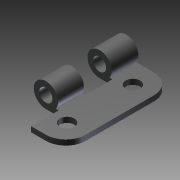
# Autodesk Inventor part: SHHPS5-2-pin
Saved by Autodesk Inventor 2015 SP1 (Build 190203100, 203)
## iProperties
Category: PARTsolutions
Company: MISUMI
Created: 2015-01-26
Part Number: SHHPS5-2-pin
Catalog Web Link: www.cadenas.de
Description: SHHPS,SHHPSD, SHHPT-pin-Stainless Steel Hinges, Steel Hinges
Vendor: MISUMI
Document SubType Name: Modeling
Designer: PARTuser1
Manufacturer: MISUMI
Mass: 1.95917 g
Surface Area: 22.9373 cm^2
Volume: 1.95917 cm^3
Density: 1 g/cm^3
Material: Generic
Appearance: PSOLRGB-192-192-192
PSOL_IDENT_0: {\\10.0.0.236\data_v8\23d-libs\misumi\metric\39_accessories_for_al_extrusions\shhps_r.prj},194 {VTYP=
PSOL_IDENT_1: 3D},{NB=SHHPS5-2-pin},{LINA=SHHPS5-2-pin},{NN=SHHPS,SHHPSD, SHHPT-pin},{DATE=17.11.2014 05:31:35},{G
PSOL_IDENT_2: EOMDATE=13.05.2009 09:15:00},{VERSION=},{LINEID=10},{LINESUBID=-1},{WBVAR=TS,NOH,ALT1}  {NB=SHHPS5-2
PSOL_IDENT_3: -pin},{LINA=SHHPS5-2-pin},{KT=DUMMY},{PN=SHHPS5-2},{TYPE=SHHPS},{TS=1},{MAT=316 Stainless Steel},{ST=
PSOL_IDENT_4: -},{NO=5},{NOH=2},{ALKG=9},{ALN=88},{MASS=43},{L=41},{W=36},{K=8.0},{P=25},{J=7.5},{S=21},{ND=5.5},{
PSOL_IDENT_5: NC=0.0},{T=2.0},{E=4.6},{R=4.6},{CR=7.5},{D=5},{AB=CBSST5-8},{QB=4},{ALT1=}
SUPPLIER: MISUMI
ARTICLENO: SHHPS5-2-pin
BOMINFO: SHHPS5-2-pin
CREATOR: CADENAS GmbH
Title: Hinge Side Right
Author: Misumi
Comments: Stainless Steel Hinges, Steel Hinges
Autodesk Inventor part; units mm, degrees
sketch "Sketch_1" plane through (0, 0, 0) normal (0, 0, 1) x (1, 0, 0)
  line L0 (0, -20.5) -> (0, 20.5)
  line L1 (0, 20.5) -> (4.6, 20.5)
  line L2 (4.6, 20.5) -> (4.6, -20.5)
  line L3 (4.6, -20.5) -> (0, -20.5)
  line L4 (0, -20.5) -> (0, 20.5)
  constraints: 10 end point
revolve "Revolution1" add sketch "Sketch_1" angle 360 about axis through (0, -20.5, 0) along (0, -1, 0)
sketch "Sketch_2" plane through (0, 0, -4.6) normal (0, 0, 1) x (1, 0, 0)
  line L0 (0, 20.5) -> (0, -20.5)
  line L1 (0, -20.5) -> (10.5, -20.5)
  arc A0 (10.5, -20.5) -> (18, -13) centre (10.5, -13) ccw
  line L2 (18, -13) -> (18, 13)
  arc A1 (18, 13) -> (10.5, 20.5) centre (10.5, 13) ccw
  line L3 (10.5, 20.5) -> (0, 20.5)
  constraints: 8 end point, 4 point on circle, 2 centre point
extrude "Extrusion1" add sketch "Sketch_2" along normal blind 2
sketch "Sketch_3" plane through (0, 0, 0) normal (0, 0, 1) x (1, 0, 0)
  line L0 (-41, 41) -> (-41, -41)
  line L1 (-41, -41) -> (41, -41)
  line L2 (41, -41) -> (41, 41)
  line L3 (41, 41) -> (-41, 41)
  line L4 (-4.6, 20.5) -> (-4.6, 10.35)
  line L5 (-4.6, 10.35) -> (4.85, 10.35)
  line L6 (4.85, 10.35) -> (4.85, -0.2)
  line L7 (4.85, -0.2) -> (-4.6, -0.2)
  line L8 (-4.6, -0.2) -> (-4.6, -10.05)
  line L9 (-4.6, -10.05) -> (4.85, -10.05)
  line L10 (4.85, -10.05) -> (4.85, -20.5)
  line L11 (4.85, -20.5) -> (18, -20.5)
  line L12 (18, -20.5) -> (18, 20.5)
  line L13 (18, 20.5) -> (-4.6, 20.5)
  constraints: 28 end point
extrude "Extrusion2" cut sketch "Sketch_3" along normal mid plane 82
sketch "Sketch_4" plane through (0, 0, 0) normal (0, 0, 1) x (1, 0, 0)
  line L0 (0, -20.5) -> (0, 20.5)
  line L1 (0, 20.5) -> (2.5, 20.5)
  line L2 (2.5, 20.5) -> (2.5, -20.5)
  line L3 (2.5, -20.5) -> (0, -20.5)
  line L4 (0, -20.5) -> (0, 20.5)
  constraints: 10 end point
revolve "Revolution2" cut sketch "Sketch_4" angle 360 about axis through (0, -20.5, 0) along (0, -1, 0)
sketch "Sketch_5" plane through (0, 12.5, 0) normal (0, 1, 0) x (1, 0, 0)
  line L0 (10.5, 2.6) -> (10.5, 4.6)
  line L1 (10.5, 4.6) -> (13.25, 4.6)
  line L2 (13.25, 4.6) -> (13.25, 2.6)
  line L3 (13.25, 2.6) -> (10.5, 2.6)
  line L4 (10.5, 2.6) -> (10.5, 4.6)
  constraints: 10 end point
revolve "Revolution3" cut sketch "Sketch_5" angle 360 about axis through (10.5, 12.5, -2.6) along (0, 0, 1)
sketch "Sketch_7" plane through (0, -12.5, 0) normal (0, 1, 0) x (1, 0, 0)
  line L0 (10.5, 2.6) -> (10.5, 4.6)
  line L1 (10.5, 4.6) -> (13.25, 4.6)
  line L2 (13.25, 4.6) -> (13.25, 2.6)
  line L3 (13.25, 2.6) -> (10.5, 2.6)
  line L4 (10.5, 2.6) -> (10.5, 4.6)
  constraints: 10 end point
revolve "Revolution4" cut sketch "Sketch_7" angle 360 about axis through (10.5, -12.5, -2.6) along (0, 0, 1)
ref_plane "r_pin_XY" through (0, 0, 0) normal (0, 1, 0) x (1, 0, 0)
ref_plane "r_pin_YZ" through (0, 0, 0) normal (1, 0, 0) x (0, 0, -1)
ref_plane "r_pin_ZX" through (0, 0, 0) normal (0, 0, -1) x (0, 1, 0)
ref_plane "hole1r_to_bolt_XY" through (10.5, 12.5, -2.6) normal (0, 0, 1) x (1, 0, 0)
ref_plane "hole1r_to_bolt_YZ" through (10.5, 12.5, -2.6) normal (1, 0, 0) x (0, 1, 0)
ref_plane "hole1r_to_bolt_ZX" through (10.5, 12.5, -2.6) normal (0, 1, 0) x (0, 0, 1)
ref_plane "hole2r_to_bolt_XY" through (10.5, -12.5, -2.6) normal (0, 0, 1) x (1, 0, 0)
ref_plane "hole2r_to_bolt_YZ" through (10.5, -12.5, -2.6) normal (1, 0, 0) x (0, 1, 0)
ref_plane "hole2r_to_bolt_ZX" through (10.5, -12.5, -2.6) normal (0, 1, 0) x (0, 0, 1)
ref_plane "hole3r_to_bolt_XY" through (10.5, 0, -2.6) normal (0, 0, 1) x (1, 0, 0)
ref_plane "hole3r_to_bolt_YZ" through (10.5, 0, -2.6) normal (1, 0, 0) x (0, 1, 0)
ref_plane "hole3r_to_bolt_ZX" through (10.5, 0, -2.6) normal (0, 1, 0) x (0, 0, 1)
body "Solid1"
